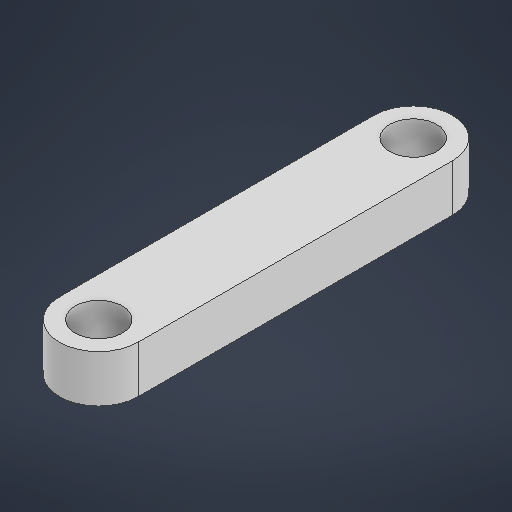
# Autodesk Inventor part: 连杆
Saved by Autodesk Inventor 2025 (Build 290162000, 162)
## iProperties
Created: 2026-04-20
Part Number: 连杆
Material: 常规
Document SubType Name: Modeling
Designer: XH
Density: 1 g/cm^3
Appearance: 默认
Author: XH
Autodesk Inventor part; units mm, degrees
ref_plane "YZ Plane" through (0, 0, 0) normal (1, 0, 0) x (0, 1, 0)
ref_plane "XZ Plane" through (0, 0, 0) normal (0, 1, 0) x (-1, 0, 0)
ref_plane "XY Plane" through (0, 0, 0) normal (0, 0, 1) x (1, 0, 0)
sketch "草图1" plane through (0, 0, 0) normal (0, 1, 0) x (-1, 0, 0)
  line L0 (0, 0) -> (0, 20) construction
  line L1 (2.5, 0) -> (2.5, 20)
  line L2 (-2.5, 20) -> (-2.5, 0)
  arc A0 (-2.5, 0) -> (2.5, 0) centre (0, 0) ccw
  arc A1 (2.5, 20) -> (-2.5, 20) centre (0, 20) ccw
  circle A2 centre (0, 0) radius 1.5
  circle A3 centre (0, 20) radius 1.5
  point P0 (0, 10)
  dimension "d0" = 2.5
  dimension "d1" = 3
  dimension "d2" = 3
  dimension "d5" = 20
  constraints: 8 end point, 4 centre point, 4 point on circle, 4 tangent, 2 coincident, 1 midpoint, 1 parallel, 1 vertical
  measures "d0" radius of A0
  measures "d1" diameter of A2
  measures "d2" diameter of A3
  measures "d5" distance of L0.start L0.end
extrude "拉伸1" add sketch "草图1" along normal blind 3
